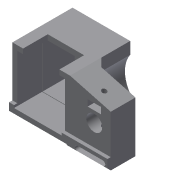
# Autodesk Inventor part: cellSTORM_UC2_motorized_micrometer_motormount
Saved by Autodesk Inventor 2019.4 (Build 234330000, 330)
## iProperties
Created: 2021-01-04
Part Number: cellSTORM_UC2_motorized_micrometer_motormount
Material: Generic
Document SubType Name: Modeling
Designer: diederichbenedict
Density: 1 g/cm^3
Appearance: Default
Author: diederichbenedict
Autodesk Inventor part; units mm, degrees
ref_plane "YZ Plane" through (0, 0, 0) normal (1, 0, 0) x (0, 1, 0)
sketch "Sketch1" plane through (0, 0, 0) normal (0, 0, 1) x (1, 0, 0)
  circle A0 centre (0, 0) radius 2.5 projected
  line L0 (11.5, 14) -> (-11.5, 14) projected
  line L1 (-17.5, -17.5) -> (17.5, -17.5)
  line L2 (17.5, -17.5) -> (17.5, 17.5)
  line L3 (17.5, 17.5) -> (-17.5, 17.5)
  line L4 (-17.5, 17.5) -> (-17.5, -17.5)
  line L5 (-17.5, -17.5) -> (17.5, 17.5) construction
  line L6 (17.5, -17.5) -> (-17.5, 17.5) construction
  circle A1 centre (32.2, 0) radius 4.725 projected
  circle A2 centre (32.2, 0) radius 4.825
  line L7 (17.5, 17.5) -> (42.2, 10.8817)
  line L8 (42.2, 10.8817) -> (42.2, 0)
  line L9 (17.5, -17.5) -> (42.2, -5.9822)
  line L10 (17.5, -17.5) -> (44.7534, -17.5) construction
  line L11 (42.2, -5.9822) -> (42.2, 0)
  line L12 (36.2709, 6.5607) -> (28.1291, 6.5607)
  line L13 (28.1291, 6.5607) -> (28.1291, 10.4571)
  line L14 (28.1291, 10.4571) -> (36.2709, 10.4571)
  line L15 (36.2709, 10.4571) -> (36.2709, 6.5607)
  line L16 (36.2709, 6.5607) -> (28.1291, 10.4571) construction
  line L17 (28.1291, 6.5607) -> (36.2709, 10.4571) construction
  point P0 (0, 0)
  point P1 (32.2, 8.5089)
  dimension "d0" = 35
  dimension "d1" = 35
  dimension "d2" = 0.1
  dimension "d3" = 25
  dimension "d4" = 75
  dimension "d5" = 10
  constraints: 34 end point, 4 midpoint, 4 parallel, 3 horizontal, 2 perpendicular, 1 centre point, 1 collinear, 1 equal length, 1 vertical
  measures "d0" distance of L3.end L2.end
  measures "d1" distance of L2.end L1.end
  measures "d2" radial gap between concentric circles of A1 A2
  measures "d3" angle of L10 L9
  measures "d4" angle of L2 L7
  measures "d5" distance from line of L11 A1.centre
extrude "Extrusion1" add sketch "Sketch1" along normal blind 3 contours L4 L3 L2 L1 | L2 L7 L8 L11 L9
sketch "Sketch2" plane through (0, 0, 0) normal (0, 0, -1) x (-1, 0, 0)
  circle A0 centre (0, 0) radius 2.5 projected
  circle A1 centre (-32.2, 0) radius 4.825 projected
  line L0 (-42.2, 10.8817) -> (-17.5, 17.5) projected
  line L1 (-42.2, -5.9822) -> (-42.2, 10.8817) projected
  line L2 (-17.5, -17.5) -> (-42.2, -5.9822) projected
  line L3 (17.5, -17.5) -> (-17.5, -17.5) projected
  line L4 (17.5, 17.5) -> (17.5, -17.5) projected
  line L5 (-17.5, 17.5) -> (17.5, 17.5) projected
  line L6 (14, 11.5) -> (14, -11.5) projected
  arc A2 (14, 11.5) -> (11.5, 14) centre (11.5, 11.5) ccw projected
  line L7 (-11.5, 14) -> (11.5, 14) projected
  arc A3 (-11.5, 14) -> (-14, 11.5) centre (-11.5, 11.5) ccw projected
  line L8 (-14, -11.5) -> (-14, 11.5) projected
  arc A4 (-14, -11.5) -> (-11.5, -14) centre (-11.5, -11.5) ccw projected
  line L9 (11.5, -14) -> (-11.5, -14) projected
  arc A5 (11.5, -14) -> (14, -11.5) centre (11.5, -11.5) ccw projected
  circle A6 centre (0, 0) radius 11 projected
  circle A7 centre (-11.5, 11.5) radius 1.025 projected
  circle A8 centre (11.5, 11.5) radius 1.025 projected
  circle A9 centre (11.5, -11.5) radius 1.025 projected
  circle A10 centre (-11.5, -11.5) radius 1.025 projected
  line L10 (-14.2, 14.2) -> (14.2, 14.2)
  line L11 (14.2, 14.2) -> (14.2, -14.2)
  line L12 (14.2, -14.2) -> (-14.2, -14.2)
  line L13 (-14.2, -14.2) -> (-14.2, 14.2)
  line L14 (-14.2, 14.2) -> (14.2, -14.2) construction
  line L15 (14.2, 14.2) -> (-14.2, -14.2) construction
  line L16 (11, 17.5) -> (-11, 17.5)
  line L17 (-11, 17.5) -> (-11, 14.2)
  line L18 (-11, 14.2) -> (11, 14.2)
  line L19 (11, 14.2) -> (11, 17.5)
  line L20 (-28.1291, 10.4571) -> (-28.1291, 6.5607) projected
  line L21 (-36.2709, 10.4571) -> (-28.1291, 10.4571) projected
  line L22 (-36.2709, 6.5607) -> (-36.2709, 10.4571) projected
  line L23 (-28.1291, 6.5607) -> (-36.2709, 6.5607) projected
  point P0 (0, 0)
  dimension "d8" = 28.4
  dimension "d9" = 28.4
  dimension "d50" = 22
  dimension "d51" = 11
  constraints: 20 end point, 4 parallel, 2 horizontal, 2 midpoint, 2 perpendicular, 2 point on line
  measures "d8" distance of L11.end L12.end
  measures "d9" distance of L10.end L11.end
  measures "d50" distance between parallel lines of L17 L19
  measures "d51" distance from line of L19 point (0, 0)
ref_plane "Work Plane1" through (26.93, -5.27, -9.3) normal (0, 0, 1) x (1, 0, 0)
extrude "Extrusion2" add sketch "Sketch2" along normal blind 12 contours L0 L5 L17 L10 L13 L12 L11 L19 L4 L3 L2 L1
sketch "Sketch3" plane through (17.5, -17.5, -12) normal (0, 0, -1) x (-1, 0, 0)
  line L0 (30.1877, 31.7) -> (31.7, 31.7) projected
  line L1 (31.7, 31.7) -> (31.7, 3.3) projected
  line L2 (31.7, 3.3) -> (3.3, 3.3) projected
  line L3 (3.3, 3.3) -> (3.3, 31.7) projected
  line L4 (3.3, 31.7) -> (5.2125, 31.7) projected
  line L5 (5.2125, 31.7) -> (5.2125, 35) projected
  line L6 (5.2125, 35) -> (0, 35) projected
  line L7 (0, 35) -> (-24.7, 28.3817) projected
  line L8 (-24.7, 28.3817) -> (-24.7, 11.5178) projected
  line L9 (-24.7, 11.5178) -> (0, 0) projected
  line L10 (0, 0) -> (35, 0) projected
  line L11 (35, 0) -> (35, 35) projected
  line L12 (35, 35) -> (30.1877, 35) projected
  line L13 (30.1877, 35) -> (30.1877, 31.7) projected
  circle A0 centre (-14.7, 17.5) radius 4.825 projected
  line L14 (0, 0) -> (0, 35)
  line L15 (5.2125, 31.7) -> (5.2125, 35) projected
  line L16 (35, 35) -> (30.1877, 35) projected
  line L17 (5.2125, 31.7) -> (30.1877, 31.7)
  line L18 (30.1877, 31.7) -> (30.1877, 35)
  line L19 (30.1877, 35) -> (5.2125, 35)
  line L20 (5.2125, 35) -> (5.2125, 31.7)
  point P0 (17.5, 17.5)
  constraints: 10 end point, 2 parallel, 1 horizontal, 1 perpendicular, 1 vertical
ref_plane "Work Plane2" through (-14, -14, -31.5) normal (0, 0, -1) x (0, 1, 0)
extrude "Extrusion3" add sketch "Sketch3" along normal up to surface (19.5 mm away) contours L13 L12 L11 L10 L14 L6 L5 L4 L3 L2 L1 L0 | L17 L5 L19 L13
sketch "Sketch4" plane through (0, 0, 3) normal (0, 0, 1) x (1, 0, 0)
  arc A0 (-13.176, 11.7849) -> (-9.9794, 10.7398) centre (-11.5, 11.5) ccw projected
  arc A1 (-12.3342, -10.0188) -> (-11.1328, -13.1599) centre (-11.5, -11.5) ccw projected
  arc A2 (10.4356, -12.8255) -> (12.904, -10.5414) centre (11.5, -11.5) ccw projected
  arc A3 (14, 11.5) -> (11.5, 14) centre (11.5, 11.5) ccw projected
  point P0 (0, 0)
hole "Hole1" at (-11.5, -11.5, 3) at (-11.5, 11.5, 3) at (11.5, 11.5, 3) at (11.5, -11.5, 3) direction (0, 0, -1) diameter 2.6 end through all
sketch "Sketch5" plane through (-17.5, -17.5, 3) normal (0, -1, 0) x (1, 0, 0)
  line L0 (54.97, -12.3) -> (54.97, -27.3)
  line L1 (44.43, -12.3) -> (44.43, -27.3)
  circle A0 centre (49.533, -6.1864) radius 1.45
  point P0 (17.5, -3)
  dimension "d21" = 2.9
  constraints: 4 end point, 2 vertical, 1 centre point, 4 other
  measures "d21" diameter of A0
extrude "Extrusion4" cut sketch "Sketch5" against normal through all
sketch "Sketch6" plane through (17.5, 17.5, -31.5) normal (0, 0, -1) x (-1, 0, 0)
  circle A0 centre (-14.7, -17.5) radius 6.65 projected
  circle A1 centre (-14.7, -17.5) radius 17.8795
  point P0 (17.5, -17.5)
  constraints: 1 centre point, 1 coincident
extrude "Extrusion5" cut sketch "Sketch6" against normal blind 15 contours A0 | A1
sketch "Sketch7" plane through (0, 0, 3) normal (0, 0, 1) x (1, 0, 0)
  circle A0 centre (11.5, 11.5) radius 1.3 projected
  circle A1 centre (-11.5, -11.5) radius 1.3 projected
  circle A2 centre (-11.5, 11.5) radius 1.3 projected
  circle A3 centre (11.5, -11.5) radius 1.3 projected
  circle A4 centre (0, 0) radius 2.5 projected
  circle A5 centre (32.2, 0) radius 4.825 projected
  line L0 (17.5, -17.5) -> (42.2, -5.9822) projected
  line L1 (42.2, -5.9822) -> (42.2, 10.8817) projected
  line L2 (42.2, 10.8817) -> (17.5, 17.5) projected
  line L3 (17.5, 17.5) -> (-17.5, 17.5) projected
  line L4 (-17.5, 17.5) -> (-17.5, -17.5) projected
  line L5 (-17.5, -17.5) -> (17.5, -17.5) projected
  line L6 (17.5, -17.5) -> (42.2, -5.9822) projected
  line L7 (42.2, -5.9822) -> (42.2, -19.9777)
  line L8 (42.2, -19.9777) -> (17.5, -19.9777)
  line L9 (17.5, -19.9777) -> (17.5, -17.5)
  line L10 (23.8963, -16.5367) -> (39.3969, -16.5367) construction
  line L11 (23.8963, -17.9867) -> (39.3969, -17.9867)
  line L12 (39.3969, -15.0867) -> (23.8963, -15.0867)
  arc A6 (23.8963, -15.0867) -> (23.8963, -17.9867) centre (23.8963, -16.5367) ccw
  arc A7 (39.3969, -17.9867) -> (39.3969, -15.0867) centre (39.3969, -16.5367) ccw
  point P0 (0, 0)
  point P1 (31.6466, -16.5367)
  dimension "d52" = 2.9
  constraints: 14 end point, 4 point on circle, 4 tangent, 2 centre point, 2 perpendicular, 1 horizontal, 1 midpoint, 1 parallel, 1 vertical
  measures "d52" diameter of A7
extrude "Extrusion6" add sketch "Sketch7" against normal up to surface (15 mm away) contours L0 L7 L8 L9
sketch "Sketch8" plane through (17.5, -17.5, -31.5) normal (0, 0, -1) x (-1, 0, 0)
  line L0 (3.3, 31.7) -> (3.3, 3.3) projected
  line L1 (31.7, 31.7) -> (3.3, 31.7) projected
  line L2 (31.7, 3.3) -> (31.7, 31.7) projected
  line L3 (3.3, 3.3) -> (31.7, 3.3) projected
  arc A0 (0, 7.3222) -> (0, 27.6778) centre (-14.7, 17.5) ccw projected
  line L4 (0, 0) -> (0, 7.3222) projected
  line L5 (35, 0) -> (0, 0) projected
  line L6 (35, 35) -> (35, 0) projected
  line L7 (0, 35) -> (35, 35) projected
  line L8 (0, 27.6778) -> (0, 35) projected
  line L9 (5.9562, 27.1005) -> (5.5467, 30.8451) projected
  circle A1 centre (6, 29) radius 1.3 projected
  circle A2 centre (29, 29) radius 1.3 projected
  arc A3 (28.4745, 5.9654) -> (27.908, 7.0484) centre (19.1062, 1.7551) ccw projected
  circle A4 centre (29, 6) radius 1.3 projected
  circle A5 centre (6, 6) radius 1.3 projected
  point P0 (17.5, 17.5)
extrude "Extrusion7" add sketch "Sketch8" along normal blind 2 contours L1 L2 L3 L0 | A0 L8 L7 L6 L5 L4
sketch "Sketch9" plane through (0, 0, 3) normal (0, 0, 1) x (1, 0, 0)
  circle A0 centre (11.5, 11.5) radius 1.3 projected
  circle A1 centre (-11.5, -11.5) radius 1.3 projected
  circle A2 centre (-11.5, 11.5) radius 1.3 projected
  circle A3 centre (11.5, -11.5) radius 1.3 projected
  circle A4 centre (0, 0) radius 2.5 projected
  circle A5 centre (32.2, 0) radius 4.825 projected
  line L0 (28.1291, 6.5607) -> (28.1291, 10.4571) projected
  line L1 (28.1291, 10.4571) -> (36.2709, 10.4571) projected
  line L2 (36.2709, 10.4571) -> (36.2709, 6.5607) projected
  line L3 (36.2709, 6.5607) -> (28.1291, 6.5607) projected
  line L4 (42.2, -19.9777) -> (42.2, 10.8817) projected
  line L5 (42.2, 10.8817) -> (17.5, 17.5) projected
  line L6 (17.5, 17.5) -> (-17.5, 17.5) projected
  line L7 (-17.5, 17.5) -> (-17.5, -17.5) projected
  line L8 (-17.5, -17.5) -> (17.5, -17.5) projected
  line L9 (42.2, 10.8817) -> (42.2, -19.9777) projected
  line L10 (42.2, -19.9777) -> (17.5, -19.9777)
  line L11 (17.5, -19.9777) -> (17.5, -12.9777)
  line L12 (17.5, -12.9777) -> (42.2, -12.9777)
  line L13 (42.2, -12.9777) -> (42.2, -19.9777)
  line L14 (17.5, -17.5) -> (17.5, -19.9777) projected
  line L15 (17.5, -19.9777) -> (42.2, -19.9777) projected
  arc A6 (39.3969, -17.9867) -> (39.3969, -15.0867) centre (39.3969, -16.5367) ccw projected
  arc A7 (23.8963, -15.0867) -> (23.8963, -17.9867) centre (23.8963, -16.5367) ccw projected
  line L16 (39.3969, -17.9867) -> (23.8963, -17.9867) projected
  line L17 (23.8963, -15.0867) -> (39.3969, -15.0867) projected
  line L18 (23.8963, -15.0867) -> (39.3969, -15.0867) projected
  line L19 (39.3969, -16.5367) -> (23.8963, -16.5367) construction
  line L20 (39.3969, -17.9867) -> (23.8963, -17.9867)
  line L21 (23.8963, -15.0867) -> (39.3969, -15.0867)
  arc A8 (39.3969, -17.9867) -> (39.3969, -15.0867) centre (39.3969, -16.5367) ccw
  arc A9 (23.8963, -15.0867) -> (23.8963, -17.9867) centre (23.8963, -16.5367) ccw
  line L22 (17.5, -12.9777) -> (-17.5, -12.9777)
  line L23 (-17.5, -12.9777) -> (-17.5, -17.5)
  line L24 (-17.5, -17.5) -> (17.5, -17.5)
  line L25 (17.5, -17.5) -> (17.5, -12.9777)
  point P0 (0, 0)
  point P1 (31.6466, -16.5367)
  dimension "d41" = 7
  constraints: 24 end point, 5 parallel, 4 point on circle, 4 tangent, 3 horizontal, 2 centre point, 2 perpendicular, 1 concentric, 1 midpoint
  measures "d41" distance of L10.end L11.end
extrude "Extrusion8" add sketch "Sketch9" along normal blind 2 contours L10 L11 L12 L4 | L11 L8 L7 L22
sketch "Sketch10" plane through (0, 0, 3) normal (0, 0, 1) x (1, 0, 0)
  line L0 (11.5, 14) -> (-11.5, 14) projected
  line L1 (11.5, -14) -> (-11.5, -14) projected
  line L2 (-14.2, -14.2) -> (-14.2, 14.2) projected
  line L3 (-11.5, -14) -> (11.5, -14) projected
  line L4 (14.2, 14.2) -> (14.2, -14.2) projected
  line L5 (14.5, -14.5) -> (-14.5, -14.5)
  line L6 (-14.5, -14.5) -> (-14.5, 14.5)
  line L7 (-14.5, 14.5) -> (14.5, 14.5)
  line L8 (14.5, 14.5) -> (14.5, -14.5)
  line L9 (14.5, -14.5) -> (-14.5, 14.5) construction
  line L10 (-14.5, -14.5) -> (14.5, 14.5) construction
  line L11 (-11, 18.1203) -> (11, 18.1203)
  line L12 (11, 18.1203) -> (11, 14.5)
  line L13 (11, 14.5) -> (-11, 14.5)
  line L14 (-11, 14.5) -> (-11, 18.1203)
  line L15 (-11, 18.1203) -> (11, 14.5) construction
  line L16 (11, 18.1203) -> (-11, 14.5) construction
  point P0 (0, 0)
  point P1 (0, 16.3101)
  dimension "d44" = 29
  dimension "d45" = 29
  dimension "d48" = 22
  dimension "d49" = 0
  constraints: 24 end point, 4 midpoint, 4 parallel, 2 horizontal, 2 perpendicular, 1 point on line
  measures "d44" distance of L6.end L7.end
  measures "d45" distance of L5.end L6.end
  measures "d48" distance between parallel lines of L12 L14
  measures "d49" horizontal distance of point (0, 0) point (0, 16.31)
extrude "Extrusion9" cut sketch "Sketch10" along normal up to surface (17 mm away) from surface at -15
chamfer "Chamfer2" distance 2 angle 45 1 edges at (29.85, -19.9777, 5)
chamfer "Chamfer3" distance 4 angle 45 1 edges at (17.5, 0, -12)
sketch "Sketch11" plane through (17.5, -17.5, -33.5) normal (0, 0, -1) x (-1, 0, 0)
  circle A0 centre (17.5, 17.5) radius 2.5 projected
  circle A1 centre (17.5, 17.5) radius 5.4635
  point P0 (17.5, 17.5)
  constraints: 1 centre point, 1 coincident
extrude "Extrusion10" cut sketch "Sketch11" against normal through all contours A0 | A1
body "Solid1"
